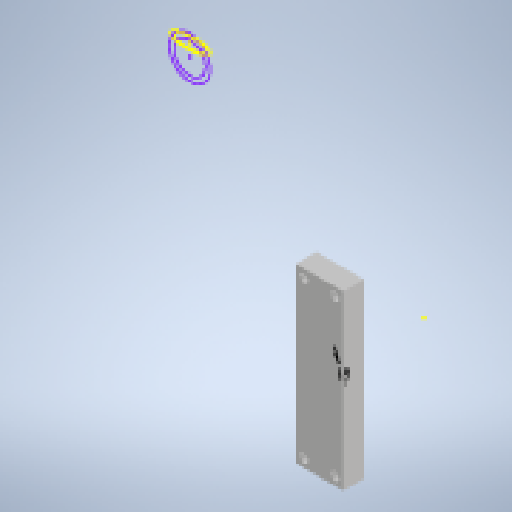
# Autodesk Inventor part: UNION_B
Saved by Autodesk Inventor 2024 (Build 280153000, 153)
## iProperties
Created: 2023-05-29
Part Number: UNION_B
Material: Genérico
Document SubType Name: Modeling
Designer: sebas
Density: 1 g/cm^3
Appearance: Valor por defecto
Mass: 28.3656 g
Surface Area: 86.854 cm^2
Volume: 28.3656 cm^3
Author: sebas
Autodesk Inventor part; units mm, degrees
ref_plane "YZ Plane" through (0, 0, 0) normal (1, 0, 0) x (0, 1, 0)
ref_plane "XZ Plane" through (0, 0, 0) normal (0, 1, 0) x (-1, 0, 0)
ref_plane "Plano de trabajo2" through (7.156, -49.9529, 91.9135) normal (-0.1189, 0.9929, 0) x (-0.9929, -0.1189, 0)
ref_plane "Plano de trabajo5" through (0, 0, 40) normal (0, 0, 1) x (1, 0, 0)
sketch "Boceto7" plane through (0, 0, 40) normal (0, 0, 1) x (1, 0, 0)
  line L0 (-7.5, 37.5) -> (7.5, 37.5)
  line L1 (7.5, 37.5) -> (7.5, -37.5)
  line L2 (7.5, -37.5) -> (-7.5, -37.5)
  line L3 (-7.5, -37.5) -> (-7.5, 37.5)
  line L4 (-7.5, 37.5) -> (7.5, -37.5) construction
  line L5 (7.5, 37.5) -> (-7.5, -37.5) construction
  line L6 (-11.5, 41.5) -> (11.5, 41.5)
  line L7 (11.5, 41.5) -> (11.5, -41.5)
  line L8 (11.5, -41.5) -> (-11.5, -41.5)
  line L9 (-11.5, -41.5) -> (-11.5, 41.5)
  line L10 (-11.5, 41.5) -> (11.5, -41.5) construction
  line L11 (11.5, 41.5) -> (-11.5, -41.5) construction
  point P0 (0, 0)
  dimension "d18" = 15
  dimension "d19" = 75
  dimension "d32" = 23
  dimension "d33" = 83
  constraints: 24 end point, 4 midpoint, 4 parallel, 2 horizontal, 2 perpendicular
  measures "d18" distance of L1.end L2.end
  measures "d19" distance of L0.end L1.end
  measures "d32" distance of L7.end L8.end
  measures "d33" distance of L6.end L7.end
extrude "Extrusión5" add sketch "Boceto7" along normal blind 10 contours L0 L1 L2 L3 | L6 L7 L8 L9
ref_plane "Plano de trabajo4" through (0, 0, 40) normal (0, 0, 1) x (1, 0, 0)
sketch "Boceto10" plane through (0, 0, 50) normal (0, 0, 1) x (1, 0, 0)
  line L0 (7.5, -37.5) -> (7.5, 37.5) projected
  line L1 (7.5, 37.5) -> (0, 37.5)
  line L2 (7.5, 37.5) -> (-7.5, 37.5) projected
  line L3 (3.75, 37.5) -> (3.75, 37.5)
  line L4 (0, 37.5) -> (0, 32.43)
  line L5 (0, 0) -> (7.5, 0)
  line L6 (0, 37.5) -> (7.5, 37.5)
  circle A0 centre (7.5, 37.5) radius 2.022
  circle A1 centre (-7.5, 37.5) radius 2.022
  circle A2 centre (7.5, -37.5) radius 2.022
  circle A3 centre (-7.5, -37.5) radius 2.022
  dimension "d28" = 0
  dimension "d35" = 7.5
  dimension "d36" = 4.044
  dimension "d37" = 4.044
  constraints: 10 end point, 4 centre point, 3 midpoint, 2 coincident, 2 symmetric about line, 1 collinear, 1 perpendicular, 1 vertical, 2 other
  measures "d28" distance of L3.start L3.end
  measures "d35" distance of L1.end L0.end
  measures "d36" diameter of A0
  measures "d37" diameter of A1
extrude "Extrusión6" cut sketch "Boceto10" against normal blind 8
sketch "Boceto11" plane through (0, 0, 40) normal (0, 0, -1) x (-1, 0, 0)
  circle A0 centre (0, 0) radius 10
  dimension "d38" = 20
  constraints: 1 centre point, 1 coincident
  measures "d38" diameter of A0
extrude "Extrusión7" add sketch "Boceto11" along normal blind 40
